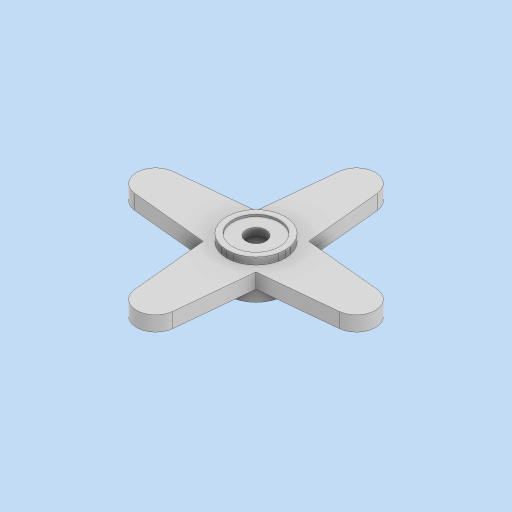
# Autodesk Inventor part: helice_cruz_mockup
Saved by Autodesk Inventor 2024 (Build 280153000, 153)
## iProperties
Created: 2024-08-28
Part Number: helice_cruz_mockup
Material: Generic
Document SubType Name: Modeling
Designer: MxMon
Density: 1 g/cm^3
Appearance: Default
Author: MxMon
Autodesk Inventor part; units mm, degrees
ref_plane "YZ Plane" through (0, 0, 0) normal (1, 0, 0) x (0, 1, 0)
ref_plane "XZ Plane" through (0, 0, 0) normal (0, 1, 0) x (-1, 0, 0)
ref_plane "XY Plane" through (0, 0, 0) normal (0, 0, 1) x (1, 0, 0)
sketch "Sketch1" plane through (0, 0, 0) normal (0, 1, 0) x (-1, 0, 0)
  circle A0 centre (0, 0) radius 2.925
  line L0 (0, 10.1) -> (0, -10.1) construction
  arc A1 (1.9158, 10.2879) -> (-1.9158, 10.2879) centre (0, 10.1) ccw
  arc A2 (-1.9158, -10.2879) -> (1.9158, -10.2879) centre (0, -10.1) ccw
  line L1 (10.1, 0) -> (-10.1, 0) construction
  arc A3 (10.2879, -1.9158) -> (10.2879, 1.9158) centre (10.1, 0) ccw
  arc A4 (-10.2879, 1.9158) -> (-10.2879, -1.9158) centre (-10.1, 0) ccw
  line L2 (1.9158, 10.2879) -> (2.925, 0)
  line L3 (-1.9158, 10.2879) -> (-2.925, 0)
  line L4 (-2.925, 0) -> (-1.9158, -10.2879)
  line L5 (2.925, 0) -> (1.9158, -10.2879)
  line L6 (10.2879, 1.9158) -> (0, 2.925)
  line L7 (10.2879, -1.9158) -> (0, -2.925)
  line L8 (-10.2879, 1.9158) -> (0, 2.925)
  line L9 (-10.2879, -1.9158) -> (0, -2.925)
  point P0 (2.6637, 2.6637)
  point P1 (-2.6637, 2.6637)
  point P2 (-2.6637, -2.6637)
  point P3 (2.6637, -2.6637)
  point P4 (-0.5684, -2.8692)
  point P5 (0.5684, -2.8692)
  point P6 (2.8692, -0.5684)
  point P7 (2.8692, 0.5684)
  point P8 (0.5684, 2.8692)
  point P9 (-0.5684, 2.8692)
  point P10 (-2.8692, 0.5684)
  point P11 (-2.8692, -0.5684)
  dimension "d0" = 5.85
  dimension "d1" = 20.2
  dimension "d2" = 3.85
  dimension "d3" = 3.85
  dimension "d4" = 20.2
  constraints: 20 end point, 12 point on circle, 6 coincident, 5 centre point, 4 equal length, 4 point on line, 4 tangent, 2 midpoint, 1 equal radius, 1 horizontal, 1 parallel, 1 vertical
  measures "d0" diameter of A0
  measures "d1" distance of L0.start L0.end
  measures "d2" diameter of A1
  measures "d3" diameter of A2
  measures "d4" distance of L1.start L1.end
extrude "Extrusion1" add sketch "Sketch1" along normal blind 1.5 contours A0 L2 L6 A3 L7 L5 | A0 L6 L2 | L5 L7 A0 | A0 L8 L3 A1 L2 L6 | L7 L5 A2 L4 L9 A0 | A0 L3 L8 | L9 L4 A0 | A0 L4 L9 A4 L8 L3
extrude "Extrusion2" add sketch "Sketch1" along normal blind 2.2 and the other way blind 1.75 contours L5 A0 L7 L9 L4 L3 L8 L6 L2
sketch "Sketch2" plane through (0, -1.75, 0) normal (0, -1, 0) x (1, 0, 0)
  circle A0 centre (0, 0) radius 2.35
  dimension "d14" = 4.7
  constraints: 1 centre point, 1 coincident
  measures "d14" diameter of A0
extrude "Extrusion3" cut sketch "Sketch2" against normal blind 2.95
sketch "Sketch3" plane through (0, 2.2, 0) normal (0, 1, 0) x (1, 0, 0)
  circle A0 centre (0, 0) radius 1
  dimension "d17" = 2
  constraints: 1 centre point, 1 coincident
  measures "d17" diameter of A0
extrude "Extrusion4" cut sketch "Sketch3" against normal blind 2.95
sketch "Sketch4" plane through (0, 2.2, 0) normal (0, 1, 0) x (1, 0, 0)
  circle A0 centre (0, 0) radius 1 projected
  circle A1 centre (0, 0) radius 2.35
  dimension "d20" = 4.7
  constraints: 1 centre point, 1 coincident
  measures "d20" diameter of A1
extrude "Extrusion5" cut sketch "Sketch4" against normal blind 0.2 contours A0 | A1
body "Solid1"
